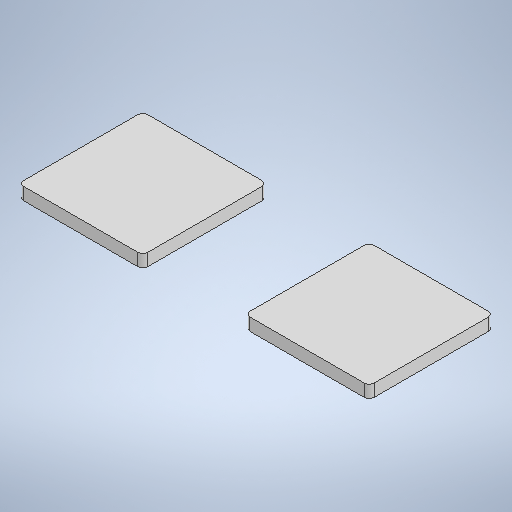
# Autodesk Inventor part: spacer
Saved by Autodesk Inventor 2025.2 (Build 292293000, 293)
## iProperties
Created: 2026-06-06
Part Number: spacer
Material: Generic
Document SubType Name: Modeling
Designer: AdminOS
Density: 1 g/cm^3
Appearance: Default
Author: AdminOS
Autodesk Inventor part; units mm, degrees
ref_plane "YZ Plane" through (0, 0, 0) normal (1, 0, 0) x (0, 1, 0)
ref_plane "XZ Plane" through (0, 0, 0) normal (0, 1, 0) x (-1, 0, 0)
ref_plane "XY Plane" through (0, 0, 0) normal (0, 0, 1) x (1, 0, 0)
sketch "Sketch1" plane through (0, 0, 0) normal (0, 1, 0) x (-1, 0, 0)
  line L0 (23, -25) -> (-23, -25)
  line L1 (-25, -23) -> (-25, 23)
  line L2 (-23, 25) -> (23, 25)
  line L3 (25, 23) -> (25, -23)
  line L4 (25, -25) -> (-25, 25) construction
  line L5 (-25, -25) -> (25, 25) construction
  line L6 (-114.1127, -25) -> (-68.1127, -25)
  line L7 (-66.1127, -23) -> (-66.1127, 23)
  line L8 (-68.1127, 25) -> (-114.1127, 25)
  line L9 (-116.1127, 23) -> (-116.1127, -23)
  line L10 (-116.1127, -25) -> (-66.1127, 25) construction
  line L11 (-66.1127, -25) -> (-116.1127, 25) construction
  arc A0 (-23, 25) -> (-25, 23) centre (-23, 23) ccw
  arc A1 (25, 23) -> (23, 25) centre (23, 23) ccw
  arc A2 (23, -25) -> (25, -23) centre (23, -23) ccw
  arc A3 (-25, -23) -> (-23, -25) centre (-23, -23) ccw
  arc A4 (-66.1127, 23) -> (-68.1127, 25) centre (-68.1127, 23) ccw
  arc A5 (-114.1127, 25) -> (-116.1127, 23) centre (-114.1127, 23) ccw
  arc A6 (-68.1127, -25) -> (-66.1127, -23) centre (-68.1127, -23) ccw
  arc A7 (-116.1127, -23) -> (-114.1127, -25) centre (-114.1127, -23) ccw
  point P0 (0, 0)
  point P1 (-91.1127, 0)
  dimension "d0" = 50
  dimension "d1" = 50
  dimension "d2" = 50
  dimension "d3" = 50
  dimension "d4" = 2
  constraints: 24 end point, 16 point on circle, 16 point on line, 16 tangent, 8 centre point, 7 equal radius, 4 midpoint, 4 parallel, 2 horizontal, 2 perpendicular
  measures "d0" distance of L4.end L5.end
  measures "d1" distance of L5.start L4.end
  measures "d2" distance of L11.end L10.end
  measures "d3" distance of L10.end L11.start
  measures "d4" radius of A0
extrude "Extrusion1" add sketch "Sketch1" along normal blind 5
body "Solid1"
